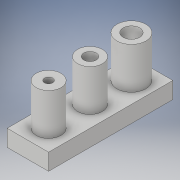
# Autodesk Inventor part: HoleSizeTest
Saved by Autodesk Inventor 2019 (Build 230136000, 136)
## iProperties
Created: 2019-05-12
Part Number: HoleSizeTest
Material: Generic
Document SubType Name: Modeling
Designer: Henry
Density: 1 g/cm^3
Appearance: Default
Author: Henry
Autodesk Inventor part; units mm, degrees
ref_plane "YZ Plane" through (0, 0, 0) normal (1, 0, 0) x (0, 1, 0)
ref_plane "XZ Plane" through (0, 0, 0) normal (0, 1, 0) x (-1, 0, 0)
ref_plane "XY Plane" through (0, 0, 0) normal (0, 0, 1) x (1, 0, 0)
sketch "Sketch1" plane through (0, 0, 0) normal (0, 1, 0) x (-1, 0, 0)
  line L0 (0, 0) -> (5, 0)
  line L1 (5, 0) -> (5, -15)
  line L2 (5, -15) -> (0, -15)
  line L3 (0, -15) -> (0, 0)
  dimension "d0" = 5
  dimension "d1" = 15
  constraints: 8 end point, 2 parallel, 1 horizontal, 1 perpendicular
  measures "d0" distance of L1.end L2.end
  measures "d1" distance of L0.end L1.end
extrude "Extrusion1" add sketch "Sketch1" along normal blind 2
sketch "Sketch2" plane through (0, 2, 0) normal (0, 1, 0) x (1, 0, 0)
  line L0 (0, 0) -> (0, 2.5)
  line L1 (0, 2.5) -> (0, 7.5)
  line L2 (0, 7.5) -> (0, 12.5)
  line L3 (0, 2.5) -> (-2.5, 2.5)
  circle A0 centre (-2.5, 2.5) radius 0.5
  circle A1 centre (-2.5, 2.5) radius 1.5
  line L4 (0, 7.5) -> (-2.5, 7.5)
  circle A2 centre (-2.5, 7.5) radius 0.75
  circle A3 centre (-2.5, 7.5) radius 1.5
  line L5 (0, 12.5) -> (-2.5, 12.5)
  circle A4 centre (-2.5, 12.5) radius 1
  circle A5 centre (-2.5, 12.5) radius 1.75
  dimension "d4" = 2.5
  dimension "d5" = 5
  dimension "d6" = 5
  dimension "d7" = 2.5
  dimension "d8" = 1
  dimension "d9" = 3
  dimension "d10" = 2.5
  dimension "d11" = 1.5
  dimension "d12" = 3
  dimension "d13" = 2.5
  dimension "d14" = 2
  dimension "d15" = 3.5
  constraints: 12 end point, 6 centre point, 6 coincident, 3 horizontal, 2 point on line, 1 vertical
  measures "d4" distance of L0.start L0.end
  measures "d5" distance of L0.end L1.end
  measures "d6" distance of L1.end L2.end
  measures "d7" distance of L0.end L3.end
  measures "d8" diameter of A0
  measures "d9" diameter of A1
  measures "d10" distance of L1.end L4.end
  measures "d11" diameter of A2
  measures "d12" diameter of A3
  measures "d13" distance of L2.end L5.end
  measures "d14" diameter of A4
  measures "d15" diameter of A5
extrude "Extrusion2" add sketch "Sketch2" along normal blind 5
body "Solid1"
